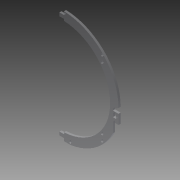
# Autodesk Inventor part: MiddleHoop
Saved by Autodesk Inventor 2013 (Build 170138000, 138)
## iProperties
Created: 2013-01-18
Part Number: MiddleHoop
Material: Polycarbonate, Clear
Document SubType Name: Modeling
Designer: motoennies
Density: 1.2 g/cm^3
Mass: 92.036 g
Surface Area: 321.94 cm^2
Volume: 76.6966 cm^3
Author: motoennies
Autodesk Inventor part; units mm, degrees
ref_plane "YZ Plane" through (0, 0, 0) normal (1, 0, 0) x (0, 1, 0)
ref_plane "XZ Plane" through (0, 0, 0) normal (0, 1, 0) x (-1, 0, 0)
ref_plane "XY Plane" through (0, 0, 0) normal (0, 0, 1) x (1, 0, 0)
sketch "Sketch1" plane through (0, 0, 0) normal (0, 0, 1) x (1, 0, 0)
  arc A0 (0, -146.05) -> (0, 146.05) centre (0, 0) ccw
  line L0 (0, 0) -> (0, 226.0912) construction
  line L1 (0, 226.0912) -> (0, -237.3269) construction
  line L2 (6.35, 145.9119) -> (6.35, 171.3324)
  line L3 (6.35, -145.9119) -> (6.35, -171.3324)
  line L4 (0, 146.05) -> (0, 151.13)
  line L5 (0, 151.13) -> (6.35, 151.13)
  line L6 (6.35, 151.13) -> (-7.62, 151.13)
  line L7 (-7.62, 151.13) -> (-7.62, 161.29)
  line L8 (-7.62, 161.29) -> (6.35, 161.29)
  line L9 (0, -146.05) -> (0, -151.13)
  line L10 (0, -151.13) -> (6.35, -151.13)
  line L11 (6.35, -151.13) -> (-7.62, -151.13)
  line L12 (-7.62, -151.13) -> (-7.62, -161.29)
  line L13 (-7.62, -161.29) -> (6.35, -161.29)
  line L14 (171.45, 0) -> (171.45, -69.85)
  line L15 (171.45, -69.85) -> (156.5761, -69.85)
  arc A1 (0, -171.45) -> (156.5761, -69.85) centre (0, 0) ccw
  arc A2 (171.45, 0) -> (0, 171.45) centre (0, 0) ccw
  dimension "d62" = 0
  dimension "d20" = 292.1
  dimension "d21" = 6.35
  dimension "d22" = 6.35
  dimension "d23" = 5.08
  dimension "d24" = 13.97
  dimension "d25" = 10.16
  dimension "d26" = 5.08
  dimension "d27" = 13.97
  dimension "d28" = 10.16
  dimension "d29" = 69.85
  dimension "d45" = 171.45
  dimension "d46" = 171.45
  constraints: 32 end point, 11 point on line, 10 point on circle, 8 perpendicular, 3 centre point, 3 collinear, 3 vertical, 1 coincident, 1 parallel, 1 tangent
  measures "d20" diameter of A0
  measures "d21" distance between parallel lines of L0 L2
  measures "d22" distance between parallel lines of L1 L3
  measures "d23" distance of L4.start L4.end
  measures "d24" distance of L5.end L6.end
  measures "d25" distance of L6.end L7.end
  measures "d26" distance of L9.start L9.end
  measures "d27" distance of L10.end L11.end
  measures "d28" distance of L11.end L12.end
  measures "d29" distance of L14.start L14.end
  measures "d45" radius of A1
  measures "d46" radius of A2
extrude "Extrusion5" add sketch "Sketch1" along normal blind 6.35 contours A0 L2 A2 L14 L15 A1 L3 | L10 L3 L13 L12 L11 | L5 L6 L7 L8 L2
sketch "Sketch3" plane through (0, 0, 6.35) normal (0, 0, 1) x (1, 0, 0)
  arc A0 (6.35, -171.3324) -> (156.5761, -69.85) centre (0, 0) ccw projected
  line L0 (156.5761, -69.85) -> (171.45, -69.85) projected
  line L1 (171.45, -69.85) -> (171.45, 0) projected
  arc A1 (171.45, 0) -> (6.35, 171.3324) centre (0, 0) ccw projected
  line L2 (6.35, 171.3324) -> (6.35, 161.29) projected
  line L3 (154.305, -22.1996) -> (154.305, -32.3596)
  line L4 (154.305, -32.3596) -> (163.83, -32.3596)
  line L5 (163.83, -32.3596) -> (163.83, -22.1996)
  line L6 (163.83, -22.1996) -> (154.305, -22.1996)
  line L7 (154.305, -15.1718) -> (171.45, -15.1718)
  line L8 (171.45, 0) -> (171.45, -15.1718)
  line L9 (154.305, -15.1718) -> (154.305, -10.0918)
  line L10 (154.305, -10.0918) -> (171.45, 0)
  line L11 (171.45, -69.85) -> (171.45, -44.45)
  line L12 (171.45, -44.45) -> (154.305, -44.45)
  line L13 (154.305, -44.45) -> (154.305, -74.7333)
  dimension "d53" = 10.16
  dimension "d54" = 9.525
  dimension "d55" = 10.16
  dimension "d56" = 37.4904
  dimension "d57" = 7.62
  dimension "d58" = 17.145
  dimension "d59" = 5.08
  dimension "d60" = 25.4
  constraints: 22 end point, 4 parallel, 3 perpendicular, 2 point on line, 1 collinear, 1 point on circle, 1 tangent
  measures "d53" distance of L3.start L3.end
  measures "d54" distance of L3.end L4.end
  measures "d55" distance of L4.end L5.end
  measures "d56" distance between parallel lines of L0 L4
  measures "d57" distance between parallel lines of L1 L5
  measures "d58" distance of L7.start L7.end
  measures "d59" distance of L7.start L9.end
  measures "d60" distance of L0.end L11.end
extrude "Extrusion7" cut sketch "Sketch3" against normal blind 25.4
sketch "Sketch4" plane through (0, 0, 6.35) normal (0, 0, 1) x (1, 0, 0)
  circle A0 centre (61.595, -163.0061) radius 3.3782 projected
  circle A1 centre (42.545, -163.0061) radius 3.3782 projected
  circle A2 centre (23.495, -163.0061) radius 3.3782 projected
  circle A3 centre (13.97, -163.0061) radius 3.3782 projected
  circle A4 centre (33.02, -163.0061) radius 3.3782 projected
  circle A5 centre (52.07, -163.0061) radius 3.3782 projected
  line L0 (7.62, -169.3561) -> (7.62, -156.6561) projected
  line L1 (66.3575, -169.3561) -> (7.62, -169.3561) projected
  line L2 (66.3575, -156.6561) -> (66.3575, -169.3561) projected
  line L3 (7.62, -156.6561) -> (66.3575, -156.6561) projected
extrude "Extrusion8" cut sketch "Sketch4" against normal blind 25.4 contours A3
sketch "Sketch5" plane through (0, 0, 6.35) normal (0, 0, 1) x (1, 0, 0)
  circle A0 centre (109.22, -93.1561) radius 3.3782 projected
  circle A1 centre (109.22, -112.2061) radius 3.3782 projected
  circle A2 centre (109.22, 94.1689) radius 3.3782 projected
  circle A3 centre (109.22, 113.2189) radius 3.3782 projected
extrude "Extrusion9" cut sketch "Sketch5" against normal blind 25.4
sketch "Sketch6" plane through (0, 0, 6.35) normal (0, 0, 1) x (1, 0, 0)
  line L0 (6.35, -161.29) -> (6.35, -171.3324) projected
  arc A0 (6.35, -171.3324) -> (154.305, -74.7333) centre (0, 0) ccw projected
  line L1 (20.32, -170.9889) -> (7.62, -170.9889) projected
  line L2 (26.4245, -169.4014) -> (6.35, -169.4014)
  dimension "d67" = 1.5875
  constraints: 2 end point, 1 perpendicular, 1 point on circle, 1 point on line
  measures "d67" distance between parallel lines of L1 L2
extrude "Extrusion10" cut sketch "Sketch6" against normal blind 25.4
body "Solid2"
